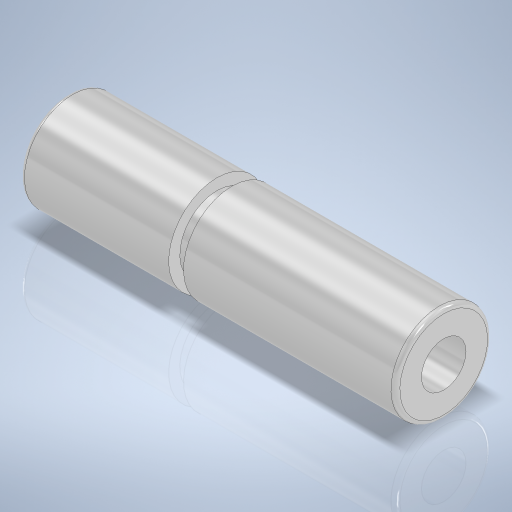
# Autodesk Inventor part: 204 Welle
Saved by Autodesk Inventor 2024 (Build 280153000, 153)
## iProperties
Created: 2024-07-12
Part Number: 204 Welle
Material: Aluminum 6061-AHC
Document SubType Name: Modeling
Designer: ffogue
Density: 2.7 g/cm^3
Appearance: Aluminium - dunkel
Author: ffogue
Autodesk Inventor part; units mm, degrees
ref_plane "YZ Plane" through (0, 0, 0) normal (1, 0, 0) x (0, 1, 0)
ref_plane "XZ Plane" through (0, 0, 0) normal (0, 1, 0) x (-1, 0, 0)
ref_plane "XY Plane" through (0, 0, 0) normal (0, 0, 1) x (1, 0, 0)
sketch "Skizze1" plane through (0, 0, 0) normal (0, 1, 0) x (-1, 0, 0)
  line L0 (0, 0) -> (0, 6.5)
  line L1 (0, 6.5) -> (-20, 6.5)
  line L2 (-20, 6.5) -> (-20, 5)
  line L3 (-20, 5) -> (-22, 5)
  line L4 (-22, 5) -> (-22, 6.5)
  line L5 (-22, 6.5) -> (-50.5, 6.5)
  line L6 (-50.5, 6.5) -> (-50.5, 0)
  line L7 (-50.5, 0) -> (0, 0)
  dimension "d0" = 13
  dimension "d1" = 20
  dimension "d2" = 2
  dimension "d3" = 28.5
  dimension "d4" = 10
  constraints: 16 end point, 6 perpendicular, 2 point on line, 1 vertical
  measures "d0" diameter of L1 L7
  measures "d1" distance between parallel lines of L2 L0
  measures "d2" distance between parallel lines of L4 L2
  measures "d3" distance between parallel lines of L6 L4
  measures "d4" diameter of L3 L7
revolve "Umdrehung1" add sketch "Skizze1" angle 360 about axis through (50.5, 0, 0) along (-1, 0, 0)
sketch "Skizze2" plane through (0, 0, 0) normal (-1, 0, 0) x (0, 0, 1)
  circle A0 centre (0, 0) radius 6.5 projected
  point P0 (0, 0)
  constraints: 1 coincident
hole "Bohrung1" at (0, 0, 0) direction (1, 0, 0) diameter 6 end through all
fillet "Rundung1" radius 0.6 2 edges at (0, 0, -6.5) (50.5, 0, -6.5)
